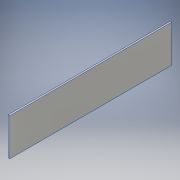
# Autodesk Inventor part: 6 x 26 x 1_4
Saved by Autodesk Inventor 2016 (Build 200138000, 138)
## iProperties
Created: 2015-06-18
Part Number: 6 x 26 x 1_4
Material: Aluminum 6061
Document SubType Name: Modeling
Designer: steele
Density: 2.7 g/cm^3
Appearance: Aluminum - Flat
Mass: 1725.56 g
Surface Area: 2116.12 cm^2
Volume: 639.095 cm^3
Author: steele
Autodesk Inventor part; units mm, degrees
ref_plane "YZ Plane" through (0, 0, 0) normal (1, 0, 0) x (0, 1, 0)
ref_plane "XZ Plane" through (0, 0, 0) normal (0, 1, 0) x (-1, 0, 0)
ref_plane "XY Plane" through (0, 0, 0) normal (0, 0, 1) x (1, 0, 0)
sketch "Sketch1" plane through (0, 0, 0) normal (1, 0, 0) x (0, 1, 0)
  line L0 (-76.2, 330.2) -> (-76.2, -330.2)
  line L1 (-76.2, -330.2) -> (76.2, -330.2)
  line L2 (76.2, -330.2) -> (76.2, 330.2)
  line L3 (76.2, 330.2) -> (-76.2, 330.2)
  line L4 (-76.2, 330.2) -> (76.2, -330.2) construction
  line L5 (-76.2, -330.2) -> (76.2, 330.2) construction
  point P0 (0, 0)
  dimension "width" = 660.4
  dimension "height" = 152.4
  constraints: 12 end point, 2 midpoint, 2 parallel, 1 perpendicular, 1 vertical
  measures "width" distance of L0.start L0.end
  measures "height" distance of L0.end L1.end
extrude "Extrusion1" add sketch "Sketch1" along normal blind 6.35
body "Solid1"
